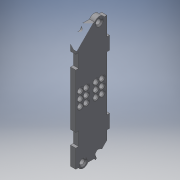
# Autodesk Inventor part: Braille cell
Saved by Autodesk Inventor 2016 (Build 200138000, 138)
## iProperties
Created: 2016-04-08
Part Number: Braille cell
Material: Generic
Document SubType Name: Modeling
Designer: Vijay
Density: 1 g/cm^3
Appearance: Default
Author: Vijay
Autodesk Inventor part; units mm, degrees
ref_plane "YZ Plane" through (0, 0, 0) normal (1, 0, 0) x (0, 1, 0)
ref_plane "XZ Plane" through (0, 0, 0) normal (0, 1, 0) x (-1, 0, 0)
ref_plane "XY Plane" through (0, 0, 0) normal (0, 0, 1) x (1, 0, 0)
sketch "Sketch1" plane through (0, 0, 0) normal (1, 0, 0) x (0, 1, 0)
  line L0 (21.6227, 12) -> (-23.4573, 12)
  line L1 (-23.4573, 12) -> (-23.4573, 0)
  line L2 (-23.4573, 0) -> (21.6227, 0)
  line L3 (21.6227, 0) -> (21.6227, 12)
  circle A0 centre (1.6227, 10.145) radius 0.95
  circle A1 centre (-0.9173, 10.145) radius 0.95
  circle A2 centre (-3.4573, 10.145) radius 0.95
  circle A3 centre (1.6227, 7.855) radius 0.95
  circle A4 centre (-0.9173, 7.855) radius 0.95
  circle A5 centre (-3.4573, 7.855) radius 0.95
  circle A6 centre (1.6227, 4.145) radius 0.95
  circle A7 centre (-0.9173, 4.145) radius 0.95
  circle A8 centre (-3.4573, 4.145) radius 0.95
  circle A9 centre (1.6227, 1.855) radius 0.95
  circle A10 centre (-0.9173, 1.855) radius 0.95
  circle A11 centre (-3.4573, 1.855) radius 0.95
  point P0 (0, 0)
  dimension "d0" = 1.9
  dimension "d3" = 2.54
  dimension "d6" = 2.29
  dimension "d11" = 6
  dimension "d18" = 1.855
  dimension "d19" = 1.855
  dimension "d32" = 20
  dimension "d33" = 20
  constraints: 12 centre point, 8 end point, 2 horizontal, 2 parallel, 2 vertical, 1 perpendicular, 22 other
  measures "d0" diameter of A0
  measures "d3" distance of A0.centre A1.centre
  measures "d6" distance of A0.centre A3.centre
  measures "d11" distance of A0.centre A6.centre
  measures "d18" distance from line of A2.centre L0
  measures "d19" distance from line of L2 A11.centre
  measures "d32" distance from line of L1 A11.centre
  measures "d33" distance from line of L3 A9.centre
extrude "Extrusion1" add sketch "Sketch1" along normal blind 2
fillet "Fillet1" radius 0.3 12 edges at (0, -4.4073, 1.855) (0, -1.8673, 1.855) (0, 0.6727, 1.855) (0, 0.6727, 4.145) (0, -4.4073, 4.145) (0, -1.8673, 4.145) (0, -4.4073, 7.855) (0, -1.8673, 7.855) (0, 0.6727, 7.855) (0, 0.6727, 10.145) (0, -1.8673, 10.145) (0, -4.4073, 10.145)
sketch "Sketch3" plane through (0, 0, 0) normal (-1, 0, 0) x (0, 0, 1)
  circle A0 centre (8.9035, 20.7205) radius 1 projected
  line L0 (6.2873, 20.7205) -> (6.9035, 20.7205) projected
  line L1 (6.2873, 8.4358) -> (6.2873, 20.7205) projected
  line L2 (7.6081, 8.4358) -> (6.2873, 8.4358) projected
  line L3 (7.6081, 8.4358) -> (7.6081, 18.7205) projected
  line L4 (7.6081, 18.7205) -> (8.2431, 18.7205) projected
  line L5 (8.2431, 6.9362) -> (8.2431, 18.7205) projected
  arc A1 (9.5639, 6.9362) -> (8.2431, 6.9362) centre (8.9035, 5.5894) ccw projected
  line L6 (9.5639, 6.9362) -> (9.5639, 18.7205) projected
  line L7 (9.5639, 18.7205) -> (10.1989, 18.7205) projected
  line L8 (10.1989, 18.7205) -> (10.1989, 8.4358) projected
  line L9 (11.5197, 8.4358) -> (10.1989, 8.4358) projected
  line L10 (11.5197, 8.4358) -> (11.5197, 20.7205) projected
  line L11 (10.9035, 20.7205) -> (11.5197, 20.7205) projected
  arc A2 (10.9035, 20.7205) -> (6.9035, 20.7205) centre (8.9035, 20.7205) ccw projected
  circle A3 centre (2.9035, 20.7205) radius 1 projected
  line L12 (0.2873, 20.7205) -> (0.9035, 20.7205) projected
  line L13 (0.2873, 20.7205) -> (0.2873, 4.4492) projected
  arc A4 (-0.1603, 2.8238) -> (0.2873, 4.4492) centre (-2.8877, 4.4492) ccw projected
  arc A5 (-0.1603, 2.8238) -> (0.1667, -0.0063) centre (1.855, 1.6227) ccw projected
  arc A6 (0.6281, -0.6175) -> (0.1667, -0.0063) centre (-2.1181, -2.2109) ccw projected
  arc A7 (0.6281, -0.6175) -> (1.6095, -1.5728) centre (2.8241, 0.6566) ccw projected
  arc A8 (1.6095, -1.5728) -> (2.3995, -0.4774) centre (1.855, -0.9173) ccw projected
  arc A9 (2.3995, -0.4774) -> (1.1594, 0.8696) centre (-6.5156, -7.4411) ccw projected
  arc A10 (1.0197, 2.2173) -> (1.1594, 0.8696) centre (1.855, 1.6227) ccw projected
  arc A11 (1.0197, 2.2173) -> (1.6081, 4.0584) centre (-1.5669, 4.0584) ccw projected
  line L14 (1.6081, 4.0584) -> (1.6081, 18.7205) projected
  line L15 (1.6081, 18.7205) -> (2.2431, 18.7205) projected
  line L16 (2.2431, 2.5029) -> (2.2431, 18.7205) projected
  arc A12 (2.0013, 2.3073) -> (2.2431, 2.5029) centre (2.0431, 2.5029) ccw projected
  arc A13 (2.0013, 2.3073) -> (1.855, 0.9227) centre (1.855, 1.6227) ccw projected
  line L17 (2.8241, 0.9227) -> (1.855, 0.9227) projected
  arc A14 (2.8241, 0.9227) -> (3.0076, 1.3568) centre (2.5666, 1.2874) ccw projected
  arc A15 (3.5176, 2.608) -> (3.0076, 1.3568) centre (4.145, 1.6227) ccw projected
  arc A16 (3.5176, 2.608) -> (3.5639, 2.6923) centre (3.4639, 2.6923) ccw projected
  line L18 (3.5639, 2.6923) -> (3.5639, 18.7205) projected
  line L19 (3.5639, 18.7205) -> (4.1989, 18.7205) projected
  line L20 (4.1989, 18.7205) -> (4.1989, 2.5108) projected
  arc A17 (4.0314, 2.3134) -> (4.1989, 2.5108) centre (3.9989, 2.5108) ccw projected
  arc A18 (4.0314, 2.3134) -> (4.145, 0.9227) centre (4.145, 1.6227) ccw projected
  line L21 (4.145, 0.9227) -> (5.2251, 0.9227) projected
  arc A19 (5.2251, 0.9227) -> (5.3226, 1.045) centre (5.2251, 1.0227) ccw projected
  arc A20 (5.4164, 2.5174) -> (5.3226, 1.045) centre (7.855, 1.6227) ccw projected
  arc A21 (5.4164, 2.5174) -> (5.5197, 3.0986) centre (3.8322, 3.0986) ccw projected
  line L22 (5.5197, 3.0986) -> (5.5197, 20.7205) projected
  line L23 (4.9035, 20.7205) -> (5.5197, 20.7205) projected
  arc A22 (4.9035, 20.7205) -> (0.9035, 20.7205) centre (2.9035, 20.7205) ccw projected
  circle A23 centre (9.0965, -22.555) radius 1 projected
  line L24 (11.7127, -22.555) -> (11.0965, -22.555) projected
  line L25 (11.7127, -22.555) -> (11.7127, -6.2837) projected
  arc A24 (12.1603, -4.6583) -> (11.7127, -6.2837) centre (14.8877, -6.2837) ccw projected
  arc A25 (12.1603, -4.6583) -> (11.8333, -1.8283) centre (10.145, -3.4573) ccw projected
  arc A26 (11.3719, -1.217) -> (11.8333, -1.8283) centre (14.1181, 0.3763) ccw projected
  arc A27 (11.3719, -1.217) -> (10.3905, -0.2617) centre (9.1759, -2.4912) ccw projected
  arc A28 (10.3905, -0.2617) -> (9.6005, -1.3571) centre (10.145, -0.9173) ccw projected
  arc A29 (9.6005, -1.3571) -> (10.8406, -2.7041) centre (18.5156, 5.6065) ccw projected
  arc A30 (10.9803, -4.0518) -> (10.8406, -2.7041) centre (10.145, -3.4573) ccw projected
  arc A31 (10.9803, -4.0518) -> (10.3919, -5.893) centre (13.5669, -5.893) ccw projected
  line L26 (10.3919, -5.893) -> (10.3919, -20.555) projected
  line L27 (10.3919, -20.555) -> (9.7569, -20.555) projected
  line L28 (9.7569, -4.3374) -> (9.7569, -20.555) projected
  arc A32 (9.9987, -4.1418) -> (9.7569, -4.3374) centre (9.9569, -4.3374) ccw projected
  arc A33 (9.9987, -4.1418) -> (10.145, -2.7573) centre (10.145, -3.4573) ccw projected
  line L29 (9.1759, -2.7573) -> (10.145, -2.7573) projected
  arc A34 (9.1759, -2.7573) -> (8.9924, -3.1913) centre (9.4334, -3.1219) ccw projected
  arc A35 (8.4824, -4.4425) -> (8.9924, -3.1913) centre (7.855, -3.4573) ccw projected
  arc A36 (8.4824, -4.4425) -> (8.4361, -4.5269) centre (8.5361, -4.5269) ccw projected
  line L30 (8.4361, -4.5269) -> (8.4361, -20.555) projected
  line L31 (8.4361, -20.555) -> (7.8011, -20.555) projected
  line L32 (7.8011, -20.555) -> (7.8011, -4.3453) projected
  arc A37 (7.9686, -4.148) -> (7.8011, -4.3453) centre (8.0011, -4.3453) ccw projected
  arc A38 (7.9686, -4.148) -> (7.855, -2.7573) centre (7.855, -3.4573) ccw projected
  line L33 (7.855, -2.7573) -> (6.7749, -2.7573) projected
  arc A39 (6.7749, -2.7573) -> (6.6774, -2.8795) centre (6.7749, -2.8573) ccw projected
  arc A40 (6.5836, -4.3519) -> (6.6774, -2.8795) centre (4.145, -3.4573) ccw projected
  arc A41 (6.5836, -4.3519) -> (6.4803, -4.9331) centre (8.1678, -4.9331) ccw projected
  line L34 (6.4803, -4.9331) -> (6.4803, -22.555) projected
  line L35 (7.0965, -22.555) -> (6.4803, -22.555) projected
  arc A42 (7.0965, -22.555) -> (11.0965, -22.555) centre (9.0965, -22.555) ccw projected
  circle A43 centre (3.0965, -22.555) radius 1 projected
  line L36 (5.7127, -22.555) -> (5.0965, -22.555) projected
  line L37 (5.7127, -22.555) -> (5.7127, -6.2837) projected
  arc A44 (6.1603, -4.6583) -> (5.7127, -6.2837) centre (8.8877, -6.2837) ccw projected
  arc A45 (6.1603, -4.6583) -> (5.8333, -1.8283) centre (4.145, -3.4573) ccw projected
  arc A46 (5.3719, -1.217) -> (5.8333, -1.8283) centre (8.1181, 0.3763) ccw projected
  arc A47 (5.3719, -1.217) -> (4.3905, -0.2617) centre (3.1759, -2.4912) ccw projected
  arc A48 (4.3905, -0.2617) -> (3.6005, -1.3571) centre (4.145, -0.9173) ccw projected
  arc A49 (3.6005, -1.3571) -> (4.8406, -2.7041) centre (12.5156, 5.6065) ccw projected
  arc A50 (4.9803, -4.0518) -> (4.8406, -2.7041) centre (4.145, -3.4573) ccw projected
  arc A51 (4.9803, -4.0518) -> (4.3919, -5.893) centre (7.5669, -5.893) ccw projected
  line L38 (4.3919, -5.893) -> (4.3919, -20.555) projected
  line L39 (4.3919, -20.555) -> (3.7569, -20.555) projected
  line L40 (3.7569, -4.3374) -> (3.7569, -20.555) projected
  arc A52 (3.9987, -4.1418) -> (3.7569, -4.3374) centre (3.9569, -4.3374) ccw projected
  arc A53 (3.9987, -4.1418) -> (4.145, -2.7573) centre (4.145, -3.4573) ccw projected
  line L41 (3.1759, -2.7573) -> (4.145, -2.7573) projected
  arc A54 (3.1759, -2.7573) -> (2.9924, -3.1913) centre (3.4334, -3.1219) ccw projected
  arc A55 (2.4824, -4.4425) -> (2.9924, -3.1913) centre (1.855, -3.4573) ccw projected
  arc A56 (2.4824, -4.4425) -> (2.4361, -4.5269) centre (2.5361, -4.5269) ccw projected
  line L42 (2.4361, -4.5269) -> (2.4361, -20.555) projected
  line L43 (2.4361, -20.555) -> (1.8011, -20.555) projected
  line L44 (1.8011, -20.555) -> (1.8011, -4.3453) projected
  arc A57 (1.9686, -4.148) -> (1.8011, -4.3453) centre (2.0011, -4.3453) ccw projected
  arc A58 (1.9686, -4.148) -> (1.855, -2.7573) centre (1.855, -3.4573) ccw projected
  line L45 (1.855, -2.7573) -> (0.7749, -2.7573) projected
  arc A59 (0.7749, -2.7573) -> (0.6774, -2.8795) centre (0.7749, -2.8573) ccw projected
  arc A60 (0.5836, -4.3519) -> (0.6774, -2.8795) centre (-1.855, -3.4573) ccw projected
  arc A61 (0.5836, -4.3519) -> (0.4803, -4.9331) centre (2.1678, -4.9331) ccw projected
  line L46 (0.4803, -4.9331) -> (0.4803, -22.555) projected
  line L47 (1.0965, -22.555) -> (0.4803, -22.555) projected
  arc A62 (1.0965, -22.555) -> (5.0965, -22.555) centre (3.0965, -22.555) ccw projected
  line L48 (0, 21.6227) -> (12, 21.6227) projected
  line L49 (12, -23.4573) -> (0, -23.4573) projected
  line L50 (10.6884, 21.6227) -> (7.1186, 21.6227)
  line L51 (0, 21.6227) -> (12, 21.6227) projected
  line L52 (4.6884, 21.6227) -> (1.1186, 21.6227)
  line L53 (12, -23.4573) -> (0, -23.4573) projected
  line L54 (10.8814, -23.4573) -> (7.3116, -23.4573)
  line L55 (4.8814, -23.4573) -> (1.3116, -23.4573)
  point P0 (0, 0)
  constraints: 8 end point, 8 point on circle, 8 point on line
extrude "Extrusion3" add sketch "Sketch3" against normal up to surface (2 mm away) contours L48 A0 | A0 L48 A2 | L48 A3 | A3 L48 A22 | L49 A23 | A23 L49 A42 | L49 A43 | A43 L49 A62 picked at (8.9035, 21.6553) picked at (2.9035, 21.6553) picked at (9.0228, -23.4816) picked at (3.0228, -23.4816)
sketch "Sketch4" plane through (0, 0, 0) normal (-1, 0, 0) x (0, 0, 1)
  circle A0 centre (8.9035, 20.7205) radius 1 projected
  circle A1 centre (2.9035, 20.7205) radius 1 projected
  circle A2 centre (9.0965, -22.555) radius 1 projected
  circle A3 centre (3.0965, -22.555) radius 1 projected
  point P0 (0, 0)
extrude "Extrusion4" cut sketch "Sketch4" against normal blind 25.4
chamfer "Chamfer1" distance 0.5 angle 45 4 edges at (2, 20.7205, 1.9035) (2, 20.7205, 7.9035) (2, -22.555, 2.0965) (2, -22.555, 8.0965)
fillet "Fillet2" radius 0.3 12 edges at (2, -4.4073, 1.855) (2, -4.4073, 4.145) (2, -1.8673, 1.855) (2, 0.6727, 1.855) (2, 0.6727, 4.145) (2, -1.8673, 4.145) (2, -1.8673, 7.855) (2, 0.6727, 7.855) (2, -4.4073, 7.855) (2, 0.6727, 10.145) (2, -1.8673, 10.145) (2, -4.4073, 10.145)
sketch "Sketch6" plane through (2, 0, 0) normal (1, 0, 0) x (0, 0, -1)
  line L0 (4.2148, -25.0355) -> (-0.05, -25.0355)
  line L1 (-0.05, -25.0355) -> (-0.05, 26.927)
  line L2 (-0.05, 26.927) -> (4.2148, 26.927)
  line L3 (4.2148, 26.927) -> (4.2148, -25.0355)
  line L4 (0, -23.4573) -> (0, 21.6227) projected
  line L5 (-21.4939, -28.5784) -> (-11.95, -28.5784)
  line L6 (-11.95, -28.5784) -> (-11.95, 24.0039)
  line L7 (-11.95, 24.0039) -> (-21.4939, 24.0039)
  line L8 (-21.4939, 24.0039) -> (-21.4939, -28.5784)
  line L9 (-12, 21.6227) -> (-12, -23.4573) projected
  point P0 (0, 0)
  dimension "d47" = 0.05
  dimension "d48" = 0.05
  constraints: 16 end point, 4 parallel, 2 horizontal, 2 perpendicular
  measures "d47" distance between parallel lines of L4 L1
  measures "d48" distance between parallel lines of L9 L6
extrude "Extrusion6" cut sketch "Sketch6" against normal blind 25.4
sketch "Sketch7" plane through (2, 0, 0) normal (1, 0, 0) x (0, 0, -1)
  line L0 (-0.05, -16.3518) -> (0.95, -16.3518)
  line L1 (0.95, -16.3518) -> (0.95, -11.3518)
  line L2 (0.95, -11.3518) -> (-0.05, -11.3518)
  line L3 (-0.05, -11.3518) -> (-0.05, -16.3518)
  line L4 (-11.95, -16.3518) -> (-10.95, -16.3518)
  line L5 (-10.95, -16.3518) -> (-10.95, -11.3518)
  line L6 (-10.95, -11.3518) -> (-11.95, -11.3518)
  line L7 (-11.95, -11.3518) -> (-11.95, -16.3518)
  line L8 (-0.05, -23.4573) -> (-0.05, 21.6227) construction
  line L9 (-0.05, -0.9173) -> (-13.7228, -0.9173) construction
  line L10 (-11.95, 21.6227) -> (-11.95, -23.4573) construction
  line L11 (-10.85, -16.4518) -> (-12.05, -16.4518)
  line L12 (-12.05, -16.4518) -> (-12.05, -11.2518)
  line L13 (-12.05, -11.2518) -> (-10.85, -11.2518)
  line L14 (-10.85, -11.2518) -> (-10.85, -16.4518)
  line L15 (-0.05, 14.5173) -> (0.95, 14.5173)
  line L16 (0.95, 14.5173) -> (0.95, 9.5173)
  line L17 (0.95, 9.5173) -> (-0.05, 9.5173)
  line L18 (-0.05, 9.5173) -> (-0.05, 14.5173)
  line L19 (-11.95, 14.5173) -> (-10.95, 14.5173)
  line L20 (-10.95, 14.5173) -> (-10.95, 9.5173)
  line L21 (-10.95, 9.5173) -> (-11.95, 9.5173)
  line L22 (-11.95, 9.5173) -> (-11.95, 14.5173)
  line L23 (-10.85, 14.6173) -> (-12.05, 14.6173)
  line L24 (-12.05, 14.6173) -> (-12.05, 9.4173)
  line L25 (-12.05, 9.4173) -> (-10.85, 9.4173)
  line L26 (-10.85, 9.4173) -> (-10.85, 14.6173)
  point P0 (0, 0)
  dimension "d51" = 1
  dimension "d52" = 1
  dimension "d53" = 5
  dimension "d54" = 0.1
  constraints: 50 end point, 12 symmetric about line, 6 parallel, 4 point on line, 3 horizontal, 3 perpendicular, 2 collinear, 1 midpoint, 3 other
  measures "d51" distance of L0.start L0.end
  measures "d52" distance of L4.start L4.end
  measures "d53" distance of L0.end L1.end
  measures "d54" distance between parallel lines of L4 L11
extrude "Extrusion7" add sketch "Sketch7" against normal up to surface (2 mm away) contours L3 L2 L1 L0 | L15 L16 L17 L18
extrude "Extrusion8" cut sketch "Sketch7" against normal blind 25.4 contours L7 L6 L5 L4 | L11 L12 L13 L14 | L19 L20 L21 L22 | L26 L25 L24 L23
body "Solid1"
